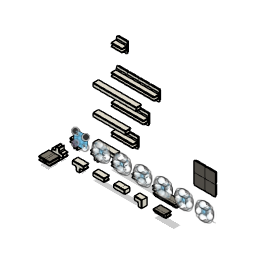
neogrid-03-master-file (Autodesk Fusion 360 design; units mm, degrees)
Autodesk Fusion 360 part; units mm, degrees
ref_plane "WorkPlane1" through (0, 0, 0) normal (0, 0, 1) x (1, 0, 0) in component "Gridfinity bin 1x1x1"
sketch "Sketch1" plane through (0, 0, 0) normal (0, 0, 1) x (1, 0, 0) in component "Gridfinity bin 1x1x1"
  line L0 (0, 0) -> (41.5, 0)
  line L1 (41.5, 0) -> (41.5, 41.5)
  line L2 (41.5, 41.5) -> (0, 41.5)
  line L3 (0, 41.5) -> (0, 0)
  dimension "d2" = 41.5
  dimension "d3" = 41.5
  constraint horizontal L0
  constraint vertical L1
  constraint horizontal L2
  constraint vertical L3
  constraint coincident L0.start L3
  constraint coincident L3.end L0
  measures "d2" horizontal distance of L0.start L0.end
  measures "d3" vertical distance of L0.end L1.end
extrude "Extrude1" add sketch "Sketch1" against normal blind 2.15 makes body 1 in component "Gridfinity bin 1x1x1"
fillet "Fillet1" radius 3.75 8 edges at (0, 0, -1.075) (41.5, 0, -1.075) (41.5, 0, -1.075) (41.5, 41.5, -1.075) (41.5, 41.5, -1.075) (0, 41.5, -1.075) (0, 41.5, -1.075) (0, 0, -1.075) on bodies 1 in component "Gridfinity bin 1x1x1"
chamfer "Chamfer1" distance 2.15 angle 45 8 edges at (1.0983, 40.4017, -2.15) (0, 20.75, -2.15) (1.0983, 1.0983, -2.15) (20.75, 0, -2.15) (40.4017, 1.0983, -2.15) (41.5, 20.75, -2.15) (40.4017, 40.4017, -2.15) (20.75, 41.5, -2.15) on bodies 1 in component "Gridfinity bin 1x1x1"
extrude "Extrude2" add 1 faces at (14.5499, 26.4167, -2.15) along direction (0, 0, -1) blind 2.6 on bodies 1 bodies 1 in component "Gridfinity bin 1x1x1"
chamfer "Chamfer2" distance 0.8 angle 45 8 edges at (2.6186, 38.8814, -4.75) (20.75, 39.35, -4.75) (38.8814, 38.8814, -4.75) (39.35, 20.75, -4.75) (38.8814, 2.6186, -4.75) (20.75, 2.15, -4.75) (2.6186, 2.6186, -4.75) (2.15, 20.75, -4.75) on bodies 1 in component "Gridfinity bin 1x1x1"
pattern_linear "R-Pattern1" count 1 spacing 42 along (1, 0, 0) of bodies 1 merged in component "Gridfinity bin 1x1x1"
sketch "Sketch2" plane through (0, 0, 0) normal (0, 0, 1) x (1, 0, 0) in component "Gridfinity bin 1x1x1"
  line L0 (0, 0) -> (41.5, 0)
  line L1 (41.5, 0) -> (41.5, 41.5)
  line L2 (41.5, 41.5) -> (0, 41.5)
  line L3 (0, 41.5) -> (0, 0)
  dimension "d16" = 41.5
  dimension "d17" = 41.5
  constraint horizontal L0
  constraint vertical L1
  constraint horizontal L2
  constraint vertical L3
  constraint coincident L0.start L3
  constraint coincident L3.end L0
  measures "d16" horizontal distance of L0.start L0.end
  measures "d17" vertical distance of L0.end L1.end
extrude "Extrude3" add sketch "Sketch2" along normal blind 2.25 separate body makes body 2 in component "Gridfinity bin 1x1x1"
fillet "Fillet2" radius 3.75 8 edges at (0, 41.5, 1.125) (41.5, 41.5, 1.125) (0, 0, 1.125) (0, 41.5, 1.125) (41.5, 41.5, 1.125) (41.5, 0, 1.125) (41.5, 0, 1.125) (0, 0, 1.125) on bodies 2 in component "Gridfinity bin 1x1x1"
combine "Combine1" operation add target body 2 tool bodies 1 1 in component "Gridfinity bin 1x1x1"
sketch "Master Dimensions" plane through (0, 0, 2.25) normal (0, 0, 1) x (1, 0, 0) in component "Gridfinity bin 1x1x1"
  arc A0 (37.75, 0) -> (41.5, 3.75) centre (37.75, 3.75) ccw
  line L0 (41.5, 3.75) -> (41.5, 37.75)
  arc A1 (41.5, 37.75) -> (37.75, 41.5) centre (37.75, 37.75) ccw
  line L1 (37.75, 41.5) -> (3.75, 41.5)
  arc A2 (3.75, 41.5) -> (0, 37.75) centre (3.75, 37.75) ccw
  line L2 (0, 37.75) -> (0, 3.75)
  arc A3 (0, 3.75) -> (3.75, 0) centre (3.75, 3.75) ccw
  line L3 (3.75, 0) -> (37.75, 0)
  line L4 (3.75, 41.5) -> (37.75, 41.5)
  line L5 (41.5, 37.75) -> (41.5, 3.75)
  line L6 (37.75, 0) -> (3.75, 0)
  line L7 (0, 3.75) -> (0, 37.75)
  arc A4 (3.75, 41.5) -> (0, 37.75) centre (3.75, 37.75) ccw
  arc A5 (41.5, 37.75) -> (37.75, 41.5) centre (37.75, 37.75) ccw
  arc A6 (0, 3.75) -> (3.75, 0) centre (3.75, 3.75) ccw
  arc A7 (37.75, 0) -> (41.5, 3.75) centre (37.75, 3.75) ccw
  line L8 (20.75, 41.5) -> (25, 41.5)
  line L9 (25, 41.5) -> (25, 0)
  line L10 (25, 0) -> (20.75, 0)
  line L11 (20.75, 0) -> (20.75, 41.5)
  line L12 (0, 20.75) -> (41.5, 20.75)
  line L13 (41.5, 20.75) -> (41.5, 25)
  line L14 (41.5, 25) -> (0, 25)
  line L15 (0, 25) -> (0, 20.75)
  line L16 (0, 20.75) -> (41.5, 20.75)
  line L17 (41.5, 20.75) -> (41.5, 16.5)
  line L18 (0, 16.5) -> (0, 20.75)
  line L19 (41.5, 16.5) -> (0, 16.5)
  line L20 (20.75, 0) -> (20.75, 41.5)
  line L21 (20.75, 41.5) -> (16.5, 41.5)
  line L22 (16.5, 0) -> (20.75, 0)
  line L23 (16.5, 41.5) -> (16.5, 0)
  line L24 (25, 41.5) -> (28, 41.5)
  line L25 (28, 41.5) -> (28, 0)
  line L26 (28, 0) -> (25, 0)
  line L27 (25, 0) -> (25, 41.5)
  line L28 (41.5, 25) -> (0, 25)
  line L29 (0, 25) -> (0, 28)
  line L30 (0, 28) -> (41.5, 28)
  line L31 (41.5, 28) -> (41.5, 25)
  line L32 (16.5, 41.5) -> (13.5, 41.5)
  line L33 (13.5, 0) -> (16.5, 0)
  line L34 (16.5, 0) -> (16.5, 41.5)
  line L35 (13.5, 41.5) -> (13.5, 0)
  line L36 (41.5, 16.5) -> (0, 16.5)
  line L37 (0, 16.5) -> (0, 13.5)
  line L38 (41.5, 13.5) -> (41.5, 16.5)
  line L39 (0, 13.5) -> (41.5, 13.5)
  line L40 (83.75, 41.5) -> (117.75, 41.5)
  arc A8 (83.75, 41.5) -> (80, 37.75) centre (83.75, 37.75) ccw
  line L41 (80, 3.75) -> (80, 37.75)
  arc A9 (80, 3.75) -> (83.75, 0) centre (83.75, 3.75) ccw
  line L42 (117.75, 0) -> (83.75, 0)
  arc A10 (117.75, 0) -> (121.5, 3.75) centre (117.75, 3.75) ccw
  line L43 (121.5, 37.75) -> (121.5, 3.75)
  arc A11 (121.5, 37.75) -> (117.75, 41.5) centre (117.75, 37.75) ccw
  line L44 (80, 28) -> (121.5, 28)
  line L45 (121.5, 25) -> (80, 25)
  line L46 (80, 20.75) -> (121.5, 20.75)
  line L47 (121.5, 16.5) -> (80, 16.5)
  line L48 (80, 13.5) -> (121.5, 13.5)
  line L49 (108, 41.5) -> (108, 0)
  line L50 (105, 41.5) -> (105, 0)
  line L51 (100.75, 0) -> (100.75, 41.5)
  line L52 (96.5, 41.5) -> (96.5, 0)
  line L53 (93.5, 41.5) -> (93.5, 0)
  line L54 (163.75, 41.5) -> (197.75, 41.5)
  arc A12 (163.75, 41.5) -> (160, 37.75) centre (163.75, 37.75) ccw
  line L55 (160, 3.75) -> (160, 37.75)
  arc A13 (160, 3.75) -> (163.75, 0) centre (163.75, 3.75) ccw
  line L56 (197.75, 0) -> (163.75, 0)
  arc A14 (197.75, 0) -> (201.5, 3.75) centre (197.75, 3.75) ccw
  line L57 (201.5, 37.75) -> (201.5, 3.75)
  arc A15 (201.5, 37.75) -> (197.75, 41.5) centre (197.75, 37.75) ccw
  line L58 (160, 28) -> (201.5, 28)
  line L59 (201.5, 25) -> (160, 25)
  line L60 (160, 20.75) -> (201.5, 20.75)
  line L61 (201.5, 16.5) -> (160, 16.5)
  line L62 (160, 13.5) -> (201.5, 13.5)
  line L63 (188, 41.5) -> (188, 0)
  line L64 (185, 41.5) -> (185, 0)
  line L65 (180.75, 0) -> (180.75, 41.5)
  line L66 (176.5, 41.5) -> (176.5, 0)
  line L67 (173.5, 41.5) -> (173.5, 0)
  line L68 (243.75, 41.5) -> (277.75, 41.5)
  arc A16 (243.75, 41.5) -> (240, 37.75) centre (243.75, 37.75) ccw
  line L69 (240, 3.75) -> (240, 37.75)
  arc A17 (240, 3.75) -> (243.75, 0) centre (243.75, 3.75) ccw
  line L70 (277.75, 0) -> (243.75, 0)
  arc A18 (277.75, 0) -> (281.5, 3.75) centre (277.75, 3.75) ccw
  line L71 (281.5, 37.75) -> (281.5, 3.75)
  arc A19 (281.5, 37.75) -> (277.75, 41.5) centre (277.75, 37.75) ccw
  line L72 (240, 28) -> (281.5, 28)
  line L73 (281.5, 25) -> (240, 25)
  line L74 (240, 20.75) -> (281.5, 20.75)
  line L75 (281.5, 16.5) -> (240, 16.5)
  line L76 (240, 13.5) -> (281.5, 13.5)
  line L77 (268, 41.5) -> (268, 0)
  line L78 (265, 41.5) -> (265, 0)
  line L79 (260.75, 0) -> (260.75, 41.5)
  line L80 (256.5, 41.5) -> (256.5, 0)
  line L81 (253.5, 41.5) -> (253.5, 0)
  line L82 (323.75, 41.5) -> (357.75, 41.5)
  arc A20 (323.75, 41.5) -> (320, 37.75) centre (323.75, 37.75) ccw
  line L83 (320, 3.75) -> (320, 37.75)
  arc A21 (320, 3.75) -> (323.75, 0) centre (323.75, 3.75) ccw
  line L84 (357.75, 0) -> (323.75, 0)
  arc A22 (357.75, 0) -> (361.5, 3.75) centre (357.75, 3.75) ccw
  line L85 (361.5, 37.75) -> (361.5, 3.75)
  arc A23 (361.5, 37.75) -> (357.75, 41.5) centre (357.75, 37.75) ccw
  line L86 (320, 28) -> (361.5, 28)
  line L87 (361.5, 25) -> (320, 25)
  line L88 (320, 20.75) -> (361.5, 20.75)
  line L89 (361.5, 16.5) -> (320, 16.5)
  line L90 (320, 13.5) -> (361.5, 13.5)
  line L91 (348, 41.5) -> (348, 0)
  line L92 (345, 41.5) -> (345, 0)
  line L93 (340.75, 0) -> (340.75, 41.5)
  line L94 (336.5, 41.5) -> (336.5, 0)
  line L95 (333.5, 41.5) -> (333.5, 0)
  line L96 (403.75, 41.5) -> (437.75, 41.5)
  arc A24 (403.75, 41.5) -> (400, 37.75) centre (403.75, 37.75) ccw
  line L97 (400, 3.75) -> (400, 37.75)
  arc A25 (400, 3.75) -> (403.75, 0) centre (403.75, 3.75) ccw
  line L98 (437.75, 0) -> (403.75, 0)
  arc A26 (437.75, 0) -> (441.5, 3.75) centre (437.75, 3.75) ccw
  line L99 (441.5, 37.75) -> (441.5, 3.75)
  arc A27 (441.5, 37.75) -> (437.75, 41.5) centre (437.75, 37.75) ccw
  line L100 (400, 28) -> (441.5, 28)
  line L101 (441.5, 25) -> (400, 25)
  line L102 (400, 20.75) -> (441.5, 20.75)
  line L103 (441.5, 16.5) -> (400, 16.5)
  line L104 (400, 13.5) -> (441.5, 13.5)
  line L105 (428, 41.5) -> (428, 0)
  line L106 (425, 41.5) -> (425, 0)
  line L107 (420.75, 0) -> (420.75, 41.5)
  line L108 (416.5, 41.5) -> (416.5, 0)
  line L109 (413.5, 41.5) -> (413.5, 0)
  line L110 (483.75, 41.5) -> (517.75, 41.5)
  arc A28 (483.75, 41.5) -> (480, 37.75) centre (483.75, 37.75) ccw
  line L111 (480, 3.75) -> (480, 37.75)
  arc A29 (480, 3.75) -> (483.75, 0) centre (483.75, 3.75) ccw
  line L112 (517.75, 0) -> (483.75, 0)
  arc A30 (517.75, 0) -> (521.5, 3.75) centre (517.75, 3.75) ccw
  line L113 (521.5, 37.75) -> (521.5, 3.75)
  arc A31 (521.5, 37.75) -> (517.75, 41.5) centre (517.75, 37.75) ccw
  line L114 (480, 28) -> (521.5, 28)
  line L115 (521.5, 25) -> (480, 25)
  line L116 (480, 20.75) -> (521.5, 20.75)
  line L117 (521.5, 16.5) -> (480, 16.5)
  line L118 (480, 13.5) -> (521.5, 13.5)
  line L119 (508, 41.5) -> (508, 0)
  line L120 (505, 41.5) -> (505, 0)
  line L121 (500.75, 0) -> (500.75, 41.5)
  line L122 (496.5, 41.5) -> (496.5, 0)
  line L123 (493.5, 41.5) -> (493.5, 0)
  point P0 (0, 41.5)
  point P1 (41.5, 41.5)
  dimension "d22" = 41.5
  dimension "d23" = 41.5
  dimension "d24" = 3.75
  dimension "d26" = 3.75
  dimension "d27" = 3.75
  dimension "d28" = 3.75
  dimension "d30" = 4.25
  dimension "d31" = 4.25
  dimension "d32" = 3
  dimension "d34" = 3
  dimension "d54" = 480
  dimension "d55" = 0
  constraint horizontal L4
  constraint vertical L5
  constraint horizontal L6
  constraint vertical L7
  constraint coincident P0 L4
  constraint coincident P0 L7
  constraint tangent L4 A4
  constraint tangent L7 A4
  constraint coincident P1 L4
  constraint coincident P1 L5
  constraint tangent L4 A5
  constraint tangent L5 A5
  constraint coincident origin L6
  constraint coincident origin L7
  constraint tangent L6 A6
  constraint tangent L7 A6
  constraint tangent L5 A7
  constraint tangent L6 A7
  constraint horizontal L8
  constraint vertical L9
  constraint horizontal L10
  constraint vertical L11
  constraint coincident L6 L9.end
  constraint midpoint L4 L8.start
  constraint horizontal L12
  constraint vertical L13
  constraint horizontal L14
  constraint vertical L15
  constraint midpoint L7 L12.start
  constraint symmetric L15.end L12 L16.start
  constraint symmetric L13.start L12 L16.end
  constraint symmetric L13.end L12 L17.end
  constraint symmetric L14.end L12 L18.start
  constraint symmetric L8.start L11 L20.end
  constraint symmetric L8.end L11 L21.end
  constraint symmetric L9.end L11 L22.start
  constraint symmetric L10.end L11 L20.start
  constraint horizontal L24
  constraint vertical L25
  constraint horizontal L26
  constraint vertical L27
  constraint horizontal L28
  constraint vertical L29
  constraint horizontal L30
  constraint vertical L31
  constraint symmetric L8.end L20 L21.end
  constraint symmetric L20 L24.end L32.end
  constraint symmetric L20 L25.end L33.start
  constraint symmetric L20 L9.end L22.start
  constraint symmetric L12 L14.end L18.start
  constraint symmetric L12 L29.end L37.end
  constraint symmetric L12 L30.end L38.start
  measures "d22" distance of P0 origin
  measures "d23" distance of P0 P1
  measures "d24" radius of A4
  measures "d26" radius of A5
  measures "d27" radius of A6
  measures "d28" radius of A7
  measures "d30" distance of L8.start L8.end
  measures "d31" distance of L12.start L14.end
  measures "d32" distance of L8.end L24.end
  measures "d34" distance of L13.end L30.end
pattern_linear "R-Pattern2" count 7 spacing 80 along (1, 0, 0) of bodies 2 makes body 3 at (105.1667, 15.0833, 2.25) makes body 4 at (185.1667, 15.0833, 2.25) makes body 5 at (265.1667, 15.0833, 2.25) makes body 6 at (345.1667, 15.0833, 2.25) makes body 7 at (425.1667, 15.0833, 2.25) makes body 8 at (505.1667, 15.0833, 2.25) in component "Gridfinity bin 1x1x1"
extrude "Extrude4" add sketch "Master Dimensions" along normal blind 21 contours L3 L6 L9 L25 L26 L27 L39 | L0 L5 L19 L25 L36 L38 L39 | L9 L19 L25 L27 L36 L39 | L3 L6 L23 L33 L34 L35 L39 | L0 L5 L14 L25 L28 L30 L31 | L19 L23 L34 L35 L36 L39 | L9 L14 L25 L27 L28 L30 | L2 L7 L19 L35 L36 L37 L39 | L1 L4 L9 L24 L25 L27 L30 | L14 L23 L28 L30 L34 L35 | L2 L7 L14 L28 L29 L30 L35 | L1 L4 L23 L30 L32 L34 L35 | L41 L44 L45 L53 | L44 L45 L52 L53 | L44 L45 L51 L52 | L44 L45 L50 L51 | L44 L45 L49 L50 | L41 L47 L48 L53 | L47 L48 L52 L53 | L43 L44 L45 L49 | L42 L48 L52 L53 | L47 L48 L49 L50 | L43 L47 L48 L49 | L42 L48 L49 L50 | L55 L58 L59 L67 | L58 L59 L66 L67 | L58 L59 L65 L66 | L58 L59 L64 L65 | L58 L59 L63 L64 | L55 L61 L62 L67 | L61 L62 L66 L67 | L57 L58 L59 L63 | L61 L62 L65 L66 | L61 L62 L64 L65 | L61 L62 L63 L64 | L57 L61 L62 L63 | L69 L72 L73 L81 | L72 L73 L80 L81 | L72 L73 L79 L80 | L72 L73 L78 L79 | L72 L73 L77 L78 | L69 L75 L76 L81 | L75 L76 L80 L81 | L71 L72 L73 L77 | L73 L74 L77 L78 | L75 L76 L79 L80 | L71 L73 L74 L77 | L74 L75 L77 L78 | L75 L76 L78 L79 | L71 L74 L75 L77 | L75 L76 L77 L78 | L71 L75 L76 L77 | L83 L86 L87 L95 | L86 L87 L94 L95 | L86 L87 L93 L94 | L86 L87 L92 L93 | L86 L87 L91 L92 | L83 L89 L90 L95 | L89 L90 L94 L95 | L87 L88 L91 L92 | L84 L90 L94 L95 | L88 L89 L91 L92 | L89 L90 L91 L92 | L84 L90 L91 L92 bodies 2 3 4 5 6 in component "Gridfinity bin 1x1x1"
chamfer "Chamfer3" distance 3 angle 45 4 edges at (28, 13.5, 12.75) (13.5, 13.5, 12.75) (28, 28, 12.75) (13.5, 28, 12.75) on bodies 2 3 6 in component "Gridfinity bin 1x1x1"
chamfer "Chamfer3" distance 3 angle 45 3 edges at (333.5, 13.5, 12.75) (108, 13.5, 12.75) (93.5, 13.5, 12.75) on bodies 2 3 6 in component "Gridfinity bin 1x1x1"
chamfer "Chamfer4" distance 3 angle 45 12 edges at (29.5, 12, 2.25) (36.25, 13.5, 2.25) (28, 5.25, 2.25) (5.25, 13.5, 2.25) (12, 12, 2.25) (13.5, 5.25, 2.25) (13.5, 36.25, 2.25) (12, 29.5, 2.25) (5.25, 28, 2.25) (36.25, 28, 2.25) (29.5, 29.5, 2.25) (28, 36.25, 2.25) on bodies 2 3 4 5 6 in component "Gridfinity bin 1x1x1"
chamfer "Chamfer4" distance 3 angle 45 16 edges at (260.75, 13.5, 2.25) (260.75, 28, 2.25) (332, 12, 2.25) (325.25, 13.5, 2.25) (333.5, 5.25, 2.25) (334, 28, 2.25) (348, 14, 2.25) (85.25, 13.5, 2.25) (116.25, 13.5, 2.25) (109.5, 12, 2.25) (108, 5.25, 2.25) (92, 12, 2.25) (93.5, 5.25, 2.25) (100.75, 28, 2.25) (180.75, 28, 2.25) (180.75, 13.5, 2.25) on bodies 2 3 4 5 6 in component "Gridfinity bin 1x1x1"
chamfer "Chamfer5" distance 1.5 angle 45 12 edges at (5.25, 13.5, 23.25) (12, 12, 23.25) (13.5, 5.25, 23.25) (28, 5.25, 23.25) (29.5, 12, 23.25) (36.25, 13.5, 23.25) (36.25, 28, 23.25) (29.5, 29.5, 23.25) (28, 36.25, 23.25) (12, 29.5, 23.25) (13.5, 36.25, 23.25) (5.25, 28, 23.25) on bodies 2 3 4 5 6 in component "Gridfinity bin 1x1x1"
chamfer "Chamfer5" distance 1.5 angle 45 17 edges at (260.75, 28, 23.25) (281.5, 20.75, 23.25) (260.75, 13.5, 23.25) (334, 28, 23.25) (348, 14, 23.25) (333.5, 5.25, 23.25) (332, 12, 23.25) (325.25, 13.5, 23.25) (85.25, 13.5, 23.25) (92, 12, 23.25) (93.5, 5.25, 23.25) (109.5, 12, 23.25) (116.25, 13.5, 23.25) (108, 5.25, 23.25) (100.75, 28, 23.25) (180.75, 28, 23.25) (180.75, 13.5, 23.25) on bodies 2 3 4 5 6 in component "Gridfinity bin 1x1x1"
extrude "Extrude5" add sketch "Master Dimensions" 1 faces at (99.3333, 22.1667, 2.25) along normal blind 21 from surface at 70 separate body contours L3 L6 L9 L25 L26 L27 L39 | L0 L5 L19 L25 L36 L38 L39 | L3 L6 L9 L10 L11 L20 L27 L39 | L9 L19 L25 L27 L36 L39 | L0 L5 L12 L16 L17 L19 L25 L36 | L3 L6 L11 L20 L22 L23 L34 L39 | L9 L11 L19 L20 L27 L36 L39 | L9 L12 L16 L19 L25 L27 L36 | L0 L5 L12 L13 L14 L16 L25 L28 | L3 L6 L23 L33 L34 L35 L39 | L11 L19 L20 L23 L34 L36 L39 | L9 L11 L12 L16 L19 L20 L27 L36 | L9 L12 L14 L16 L25 L27 L28 | L0 L5 L14 L25 L28 L30 L31 | L19 L23 L34 L35 L36 L39 | L11 L12 L16 L19 L20 L23 L34 L36 | L9 L11 L12 L14 L16 L20 L27 L28 | L9 L14 L25 L27 L28 L30 | L2 L7 L19 L35 L36 L37 L39 | L12 L16 L19 L23 L34 L35 L36 | L11 L12 L14 L16 L20 L23 L28 L34 | L9 L11 L14 L20 L27 L28 L30 | L1 L4 L9 L24 L25 L27 L30 | L2 L7 L12 L16 L18 L19 L35 L36 | L12 L14 L16 L23 L28 L34 L35 | L11 L14 L20 L23 L28 L30 L34 | L1 L4 L8 L9 L11 L20 L27 L30 | L2 L7 L12 L14 L15 L16 L28 L35 | L14 L23 L28 L30 L34 L35 | L1 L4 L11 L20 L21 L23 L30 L34 | L2 L7 L14 L28 L29 L30 L35 | L1 L4 L23 L30 L32 L34 L35 | L41 L44 L45 L53 | L44 L45 L52 L53 | L44 L45 L51 L52 | L44 L45 L50 L51 | L44 L45 L49 L50 | L41 L47 L48 L53 | L47 L48 L52 L53 | L43 L44 L45 L49 | L42 L48 L52 L53 | L47 L48 L49 L50 | L43 L47 L48 L49 | L42 L48 L49 L50 | L55 L58 L59 L67 | L58 L59 L66 L67 | L58 L59 L65 L66 | L55 L59 L60 L67 | L59 L60 L66 L67 | L58 L59 L64 L65 | L59 L60 L65 L66 | L55 L60 L61 L67 | L60 L61 L66 L67 | L58 L59 L63 L64 | L59 L60 L64 L65 | L60 L61 L65 L66 | L55 L61 L62 L67 | L61 L62 L66 L67 | L57 L58 L59 L63 | L59 L60 L63 L64 | L60 L61 L64 L65 | L61 L62 L65 L66 | L57 L59 L60 L63 | L60 L61 L63 L64 | L61 L62 L64 L65 | L57 L60 L61 L63 | L61 L62 L63 L64 | L57 L61 L62 L63 | L69 L72 L73 L81 | L72 L73 L80 L81 | L72 L73 L79 L80 | L69 L73 L74 L81 | L73 L74 L80 L81 | L72 L73 L78 L79 | L73 L74 L79 L80 | L69 L74 L75 L81 | L74 L75 L80 L81 | L72 L73 L77 L78 | L73 L74 L78 L79 | L74 L75 L79 L80 | L69 L75 L76 L81 | L75 L76 L80 L81 | L71 L72 L73 L77 | L73 L74 L77 L78 | L74 L75 L78 L79 | L75 L76 L79 L80 | L71 L73 L74 L77 | L74 L75 L77 L78 | L75 L76 L78 L79 | L71 L74 L75 L77 | L75 L76 L77 L78 | L71 L75 L76 L77 | L83 L86 L87 L95 | L86 L87 L94 L95 | L86 L87 L93 L94 | L83 L87 L88 L95 | L87 L88 L94 L95 | L86 L87 L92 L93 | L87 L88 L93 L94 | L83 L88 L89 L95 | L88 L89 L94 L95 | L86 L87 L91 L92 | L87 L88 L92 L93 | L88 L89 L93 L94 | L83 L89 L90 L95 | L89 L90 L94 L95 | L87 L88 L91 L92 | L88 L89 L92 L93 | L89 L90 L93 L94 | L84 L90 L94 L95 | L88 L89 L91 L92 | L89 L90 L92 L93 | L84 L90 L93 L94 | L89 L90 L91 L92 | L84 L90 L92 L93 | L84 L90 L91 L92 | L97 L100 L101 L109 | L100 L101 L108 L109 | L100 L101 L107 L108 | L97 L101 L102 L109 | L101 L102 L108 L109 | L100 L101 L106 L107 | L101 L102 L107 L108 | L97 L102 L103 L109 | L102 L103 L108 L109 | L100 L101 L105 L106 | L101 L102 L106 L107 | L102 L103 L107 L108 | L97 L103 L104 L109 | L103 L104 L108 L109 | L99 L100 L101 L105 | L101 L102 L105 L106 | L102 L103 L106 L107 | L103 L104 L107 L108 | L99 L101 L102 L105 | L102 L103 L105 L106 | L103 L104 L106 L107 | L99 L102 L103 L105 | L103 L104 L105 L106 | L99 L103 L104 L105 on bodies 3 makes body 9 at (18.3333, 18.3333, 72.25) makes body 10 at (343.1667, 13.8333, 72.25) makes body 11 at (253.8333, 13.5, 86.25) makes body 12 at (93.8333, 28, 86.25) makes body 13 at (173.8333, 13.5, 86.25) makes body 14 at (413.8333, 13.5, 86.25) in component "Gridfinity bin 1x1x1"
extrude "Extrude6" cut sketch "Master Dimensions" along normal blind 18 from surface at 70 contours L3 L6 L9 L10 L11 L20 L27 L39 | L0 L5 L12 L16 L17 L19 L25 L36 | L3 L6 L11 L20 L22 L23 L34 L39 | L9 L11 L19 L20 L27 L36 L39 | L9 L12 L16 L19 L25 L27 L36 | L0 L5 L12 L13 L14 L16 L25 L28 | L11 L19 L20 L23 L34 L36 L39 | L9 L11 L12 L16 L19 L20 L27 L36 | L9 L12 L14 L16 L25 L27 L28 | L11 L12 L16 L19 L20 L23 L34 L36 | L9 L11 L12 L14 L16 L20 L27 L28 | L12 L16 L19 L23 L34 L35 L36 | L11 L12 L14 L16 L20 L23 L28 L34 | L9 L11 L14 L20 L27 L28 L30 | L2 L7 L12 L16 L18 L19 L35 L36 | L12 L14 L16 L23 L28 L34 L35 | L11 L14 L20 L23 L28 L30 L34 | L1 L4 L8 L9 L11 L20 L27 L30 | L2 L7 L12 L14 L15 L16 L28 L35 | L1 L4 L11 L20 L21 L23 L30 L34 | L41 L45 L46 L53 | L45 L46 L52 L53 | L45 L46 L51 L52 | L41 L46 L47 L53 | L46 L47 L52 L53 | L45 L46 L50 L51 | L46 L47 L51 L52 | L45 L46 L49 L50 | L46 L47 L50 L51 | L47 L48 L51 L52 | L43 L45 L46 L49 | L46 L47 L49 L50 | L47 L48 L50 L51 | L42 L48 L51 L52 | L43 L46 L47 L49 | L42 L48 L50 L51 | L55 L59 L60 L67 | L59 L60 L66 L67 | L59 L60 L65 L66 | L55 L60 L61 L67 | L60 L61 L66 L67 | L59 L60 L64 L65 | L60 L61 L65 L66 | L59 L60 L63 L64 | L60 L61 L64 L65 | L57 L59 L60 L63 | L60 L61 L63 L64 | L57 L60 L61 L63 | L69 L73 L74 L81 | L73 L74 L80 L81 | L73 L74 L79 L80 | L69 L74 L75 L81 | L74 L75 L80 L81 | L73 L74 L78 L79 | L74 L75 L79 L80 | L74 L75 L78 L79 | L83 L87 L88 L95 | L87 L88 L94 L95 | L87 L88 L93 L94 | L83 L88 L89 L95 | L88 L89 L94 L95 | L87 L88 L92 L93 | L88 L89 L93 L94 | L88 L89 L92 L93 | L89 L90 L93 L94 | L89 L90 L92 L93 | L84 L90 L93 L94 | L84 L90 L92 L93 | L97 L101 L102 L109 | L101 L102 L108 L109 | L101 L102 L107 L108 | L97 L102 L103 L109 | L102 L103 L108 L109 | L101 L102 L106 L107 | L102 L103 L107 L108 | L101 L102 L105 L106 | L102 L103 L106 L107 | L99 L101 L102 L105 | L102 L103 L105 L106 | L99 L102 L103 L105 bodies 14 9 13 10 12 11 in component "Gridfinity bin 1x1x1"
chamfer "Chamfer6" distance 3 angle 45 4 edges at (28, 28, 82.75) (13.5, 28, 82.75) (13.5, 13.5, 82.75) (28, 13.5, 82.75) on bodies 9 10 12 in component "Gridfinity bin 1x1x1"
chamfer "Chamfer6" distance 3 angle 45 3 edges at (333.5, 13.5, 82.75) (108, 13.5, 82.75) (93.5, 13.5, 82.75) on bodies 9 10 12 in component "Gridfinity bin 1x1x1"
chamfer "Chamfer7" distance 1.5 angle 45 12 edges at (13.5, 36.25, 93.25) (12, 29.5, 93.25) (5.25, 28, 93.25) (5.25, 13.5, 93.25) (12, 12, 93.25) (13.5, 5.25, 93.25) (28, 5.25, 93.25) (29.5, 12, 93.25) (36.25, 13.5, 93.25) (36.25, 28, 93.25) (29.5, 29.5, 93.25) (28, 36.25, 93.25) on bodies 9 10 11 12 13 14 in component "Gridfinity bin 1x1x1"
chamfer "Chamfer7" distance 1.5 angle 45 17 edges at (180.75, 28, 93.25) (180.75, 13.5, 93.25) (334, 28, 93.25) (348, 14, 93.25) (333.5, 5.25, 93.25) (332, 12, 93.25) (325.25, 13.5, 93.25) (260.75, 28, 93.25) (260.75, 13.5, 93.25) (281.5, 20.75, 93.25) (116.25, 13.5, 93.25) (109.5, 12, 93.25) (108, 5.25, 93.25) (85.25, 13.5, 93.25) (93.5, 5.25, 93.25) (92, 12, 93.25) (100.75, 28, 93.25) on bodies 9 10 11 12 13 14 in component "Gridfinity bin 1x1x1"
chamfer "Chamfer7" distance 1.5 angle 45 1 edges at (420.75, 28, 93.25) on bodies 9 10 11 12 13 14 in component "Gridfinity bin 1x1x1"
chamfer "Chamfer8" distance 1.5 angle 45 12 edges at (28, 36.25, 72.25) (29.5, 29.5, 72.25) (36.25, 28, 72.25) (12, 29.5, 72.25) (5.25, 28, 72.25) (13.5, 36.25, 72.25) (12, 12, 72.25) (13.5, 5.25, 72.25) (5.25, 13.5, 72.25) (29.5, 12, 72.25) (36.25, 13.5, 72.25) (28, 5.25, 72.25) on bodies 9 in component "Gridfinity bin 1x1x1"
sketch "Sketch1 (2)" plane through (441.5, 0, 0) normal (1, 0, 0) x (0, 0, -1)
  line L0 (-91.75, 28) -> (-93.25, 26.5)
  line L1 (-93.25, 26.5) -> (-93.25, 13.5)
  line L2 (-93.25, 13.5) -> (-72.25, 13.5)
  line L3 (-72.25, 13.5) -> (-72.25, 16.5)
  line L4 (-72.25, 16.5) -> (-90.25, 16.5)
  line L5 (-90.25, 16.5) -> (-90.25, 25)
  line L6 (-90.25, 25) -> (-72.25, 25)
  line L7 (-72.25, 25) -> (-72.25, 28)
  line L8 (-72.25, 28) -> (-91.75, 28)
  line L9 (-93.25, 13.5) -> (-101.6216, 28)
  line L10 (-101.6216, 28) -> (-91.75, 28)
  dimension "d76" = 30
  constraint coincident L1.end L2.start
  constraint coincident L0.start L8.end
  constraint collinear L8 L10
  measures "d76" angle of L1 L9
extrude "Extrude7" add sketch "Sketch1 (2)" against normal up to surface (41.5 mm away) contours L0 L1 L9 L10 bodies 14 in component "Gridfinity bin 1x1x1"
chamfer "Chamfer9" distance 1.5 angle 45 1 edges at (420.75, 28, 101.6216) on bodies 14 in component "Gridfinity bin 1x1x1"
pattern_linear "R-Pattern3" count 2 spacing 55 along (0, 1, 0) of bodies 14 makes body 15 in component "Gridfinity bin 1x1x1"
extrude "Extrude8" add 1 faces at (441.5, 77.7337, 93.7905) along direction (1, 0, 0) blind 41.5 on bodies 15 bodies 15 in component "Gridfinity bin 1x1x1"
pattern_linear "R-Pattern4" count 5 spacing 100 along (0, 1, 0) of bodies 4 makes body 16 at (174.8165, 115.0833, -4.75) makes body 17 at (174.8165, 215.0833, -4.75) makes body 18 at (174.8165, 315.0833, -4.75) makes body 19 at (174.8165, 415.0833, -4.75) in component "Gridfinity bin 1x1x1"
pattern_linear "R-Pattern5" count 2 spacing 41.5 along (1, 0, 0) of bodies 16 makes body 20 in component "Gridfinity bin 1x1x1"
combine "Combine2" operation add target body 16 tool bodies 20 in component "Gridfinity bin 1x1x1"
sketch "Sketch3" plane through (160, 0, 0) normal (-1, 0, 0) x (0, 0, 1)
  line L0 (21.75, 113.5) -> (23.25, 115)
  line L1 (23.25, 115) -> (23.25, 116.5)
  line L2 (23.25, 116.5) -> (2.25, 116.5)
  line L3 (2.25, 116.5) -> (2.25, 125)
  line L4 (2.25, 125) -> (23.25, 125)
  line L5 (23.25, 125) -> (23.25, 126.5)
  line L6 (23.25, 126.5) -> (21.75, 128)
  line L7 (21.75, 128) -> (5.25, 128)
  line L8 (5.25, 128) -> (2.25, 131)
  line L9 (2.25, 131) -> (2.25, 137.75)
  line L10 (2.25, 137.75) -> (0, 137.75)
  line L11 (0, 137.75) -> (0, 103.75)
  line L12 (0, 103.75) -> (2.25, 103.75)
  line L13 (2.25, 103.75) -> (2.25, 110.5)
  line L14 (2.25, 110.5) -> (5.25, 113.5)
  line L15 (5.25, 113.5) -> (21.75, 113.5)
  line L16 (0, 100) -> (2.25, 100)
  line L17 (2.25, 100) -> (2.25, 141.5)
  line L18 (2.25, 141.5) -> (0, 141.5)
  line L19 (0, 141.5) -> (0, 100)
  line L20 (2.25, 141.5) -> (0, 141.5)
  line L21 (0, 100) -> (2.25, 100)
  constraint horizontal L16
  constraint vertical L17
  constraint horizontal L18
  constraint vertical L19
  constraint collinear L18 L20
  constraint collinear L16 L21
extrude "Extrude9" add sketch "Sketch3" against normal blind 30 from surface at -30 contours L12 L16 L17 L19 L21 | L10 L17 L18 L19 L20 bodies 16 in component "Gridfinity bin 1x1x1"
pattern_linear "R-Pattern6" count 3 spacing 41.5 along (1, 0, 0) of bodies 17 makes body 21 at (216.3165, 215.0833, -4.75) makes body 22 at (257.8165, 215.0833, -4.75) in component "Gridfinity bin 1x1x1"
pattern_linear "R-Pattern7" count 4 spacing 41.5 along (1, 0, 0) of bodies 18 makes body 23 at (216.3165, 315.0833, -4.75) makes body 24 at (257.8165, 315.0833, -4.75) makes body 25 at (299.3165, 315.0833, -4.75) in component "Gridfinity bin 1x1x1"
combine "Combine3" operation add target body 17 tool bodies 21 22 in component "Gridfinity bin 1x1x1"
combine "Combine4" operation add target body 18 tool bodies 23 24 25 in component "Gridfinity bin 1x1x1"
sketch "Sketch4" plane through (160, 0, 0) normal (-1, 0, 0) x (0, 0, 1)
  line L0 (21.75, 213.5) -> (23.25, 215)
  line L1 (23.25, 215) -> (23.25, 216.5)
  line L2 (23.25, 216.5) -> (2.25, 216.5)
  line L3 (2.25, 216.5) -> (2.25, 225)
  line L4 (2.25, 225) -> (23.25, 225)
  line L5 (23.25, 225) -> (23.25, 226.5)
  line L6 (23.25, 226.5) -> (21.75, 228)
  line L7 (21.75, 228) -> (5.25, 228)
  line L8 (5.25, 228) -> (2.25, 231)
  line L9 (2.25, 231) -> (2.25, 237.75)
  line L10 (2.25, 237.75) -> (0, 237.75)
  line L11 (0, 237.75) -> (0, 203.75)
  line L12 (0, 203.75) -> (2.25, 203.75)
  line L13 (2.25, 203.75) -> (2.25, 210.5)
  line L14 (2.25, 210.5) -> (5.25, 213.5)
  line L15 (5.25, 213.5) -> (21.75, 213.5)
  line L16 (0, 241.5) -> (2.25, 241.5)
  line L17 (2.25, 241.5) -> (2.25, 200)
  line L18 (2.25, 200) -> (0, 200)
  line L19 (0, 200) -> (0, 241.5)
  line L20 (0, 200) -> (2.25, 200)
  line L21 (2.25, 241.5) -> (0, 241.5)
  constraint horizontal L16
  constraint vertical L17
  constraint horizontal L18
  constraint vertical L19
  constraint collinear L3 L17
  constraint collinear L18 L20
  constraint collinear L16 L21
  constraint collinear L11 L19
extrude "Extrude10" add sketch "Sketch4" against normal blind 74 from surface at -30 contours L12 L17 L18 L19 L20 | L10 L16 L17 L19 L21 bodies 17 in component "Gridfinity bin 1x1x1"
sketch "Sketch5" plane through (160, 0, 0) normal (-1, 0, 0) x (0, 0, 1)
  line L0 (21.75, 313.5) -> (23.25, 315)
  line L1 (23.25, 315) -> (23.25, 316.5)
  line L2 (23.25, 316.5) -> (2.25, 316.5)
  line L3 (2.25, 316.5) -> (2.25, 325)
  line L4 (2.25, 325) -> (23.25, 325)
  line L5 (23.25, 325) -> (23.25, 326.5)
  line L6 (23.25, 326.5) -> (21.75, 328)
  line L7 (21.75, 328) -> (5.25, 328)
  line L8 (5.25, 328) -> (2.25, 331)
  line L9 (2.25, 331) -> (2.25, 337.75)
  line L10 (2.25, 337.75) -> (0, 337.75)
  line L11 (0, 337.75) -> (0, 303.75)
  line L12 (0, 303.75) -> (2.25, 303.75)
  line L13 (2.25, 303.75) -> (2.25, 310.5)
  line L14 (2.25, 310.5) -> (5.25, 313.5)
  line L15 (5.25, 313.5) -> (21.75, 313.5)
  line L16 (0, 341.5) -> (2.25, 341.5)
  line L17 (2.25, 341.5) -> (2.25, 300)
  line L18 (2.25, 300) -> (0, 300)
  line L19 (0, 300) -> (0, 341.5)
  line L20 (0, 300) -> (2.25, 300)
  line L21 (2.25, 341.5) -> (0, 341.5)
  constraint horizontal L16
  constraint vertical L17
  constraint horizontal L18
  constraint vertical L19
  constraint collinear L18 L20
  constraint collinear L16 L21
extrude "Extrude11" add sketch "Sketch5" against normal blind 106 from surface at -30 contours L12 L17 L18 L19 L20 | L10 L16 L17 L19 L21 bodies 18 in component "Gridfinity bin 1x1x1"
pattern_linear "R-Pattern8" count 4 spacing 100 along (0, 1, 0) of bodies 13 makes body 26 at (173.8333, 128, 78.75) makes body 27 at (173.8333, 228, 78.75) makes body 28 at (173.8333, 328, 78.75) in component "Gridfinity bin 1x1x1"
extrude "Extrude12" add 1 faces at (201.5, 127, 84.75) along direction (1, 0, 0) blind 41.5 on bodies 26 bodies 26 in component "Gridfinity bin 1x1x1"
extrude "Extrude13" add 1 faces at (201.5, 214.5, 84.75) along direction (1, 0, 0) blind 83 on bodies 27 bodies 27 in component "Gridfinity bin 1x1x1"
extrude "Extrude14" add 1 faces at (201.5, 314.5, 84.75) along direction (1, 0, 0) blind 124.5 on bodies 28 bodies 28 in component "Gridfinity bin 1x1x1"
ref_plane "WorkPlane1" through (0, 0, 0) normal (0, 0, 1) x (1, 0, 0) in component "Neogrid - Base Cover 2x2"
sketch "Sketch1 (3)" plane through (0, 0, 0) normal (0, 0, 1) x (1, 0, 0) in component "Neogrid - Base Cover 2x2"
  line L0 (0, 0) -> (41.5, 0)
  line L1 (41.5, 0) -> (41.5, 41.5)
  line L2 (41.5, 41.5) -> (0, 41.5)
  line L3 (0, 41.5) -> (0, 0)
  dimension "d113" = 41.5
  dimension "d114" = 41.5
  constraint horizontal L0
  constraint vertical L1
  constraint horizontal L2
  constraint vertical L3
  constraint coincident L0.start L3
  constraint coincident L3.end L0
  measures "d113" horizontal distance of L0.start L0.end
  measures "d114" vertical distance of L0.end L1.end
extrude "Extrude1'" add sketch "Sketch1 (3)" against normal blind 2.15 separate body makes body 29 in component "Neogrid - Base Cover 2x2"
fillet "Fillet1'" radius 3.75 8 edges at (0, 0, -1.075) (41.5, 0, -1.075) (41.5, 0, -1.075) (41.5, 41.5, -1.075) (41.5, 41.5, -1.075) (0, 41.5, -1.075) (0, 41.5, -1.075) (0, 0, -1.075) on bodies 29 in component "Neogrid - Base Cover 2x2"
chamfer "Chamfer1'" distance 2.15 angle 45 8 edges at (1.0983, 40.4017, -2.15) (0, 20.75, -2.15) (1.0983, 1.0983, -2.15) (20.75, 0, -2.15) (40.4017, 1.0983, -2.15) (41.5, 20.75, -2.15) (40.4017, 40.4017, -2.15) (20.75, 41.5, -2.15) on bodies 29 in component "Neogrid - Base Cover 2x2"
extrude "Extrude2'" add 1 faces at (14.5499, 26.4167, -2.15) along direction (0, 0, -1) blind 2.6 on bodies 29 bodies 29 in component "Neogrid - Base Cover 2x2"
chamfer "Chamfer2'" distance 0.8 angle 45 8 edges at (2.6186, 38.8814, -4.75) (20.75, 39.35, -4.75) (38.8814, 38.8814, -4.75) (39.35, 20.75, -4.75) (38.8814, 2.6186, -4.75) (20.75, 2.15, -4.75) (2.6186, 2.6186, -4.75) (2.15, 20.75, -4.75) on bodies 29 in component "Neogrid - Base Cover 2x2"
pattern_linear "R-Pattern1'" count 2 spacing 42 along (1, 0, 0) count 2 spacing 42 along (0, 1, 0) of bodies 29 makes body 30 at (68.4167, 16.3333, 0) makes body 31 at (25.1667, 57.0833, 0) makes body 32 at (68.4167, 58.3333, 0) in component "Neogrid - Base Cover 2x2"
sketch "Sketch2 (2)" plane through (0, 0, 0) normal (0, 0, 1) x (1, 0, 0) in component "Neogrid - Base Cover 2x2"
  line L0 (0, 0) -> (83.5, 0)
  line L1 (83.5, 0) -> (83.5, 83.5)
  line L2 (83.5, 83.5) -> (0, 83.5)
  line L3 (0, 83.5) -> (0, 0)
  dimension "d127" = 83.5
  dimension "d128" = 83.5
  constraint horizontal L0
  constraint vertical L1
  constraint horizontal L2
  constraint vertical L3
  constraint coincident L0.start L3
  constraint coincident L3.end L0
  measures "d127" horizontal distance of L0.start L0.end
  measures "d128" vertical distance of L0.end L1.end
extrude "Extrude3'" add sketch "Sketch2 (2)" along normal blind 2.25 separate body makes body 33 in component "Neogrid - Base Cover 2x2"
fillet "Fillet2'" radius 3.75 8 edges at (0, 83.5, 1.125) (83.5, 83.5, 1.125) (83.5, 83.5, 1.125) (83.5, 0, 1.125) (83.5, 0, 1.125) (0, 0, 1.125) (0, 0, 1.125) (0, 83.5, 1.125) on bodies 33 in component "Neogrid - Base Cover 2x2"
combine "Combine1'" operation add target body 33 tool bodies 29 30 31 32 29 in component "Neogrid - Base Cover 2x2"
move_body "Move1" bodies 33 to x (1, 0, 0) y (0, 1, 0) z (0, 0, 1) at (460, 90, 0) in component "Neogrid - Base Cover 2x2"
ref_plane "WorkPlane1" through (0, 0, 0) normal (0, 0, 1) x (1, 0, 0) in component "Neogrid - Base Cover 2x1"
sketch "Sketch1 (4)" plane through (0, 0, 0) normal (0, 0, 1) x (1, 0, 0) in component "Neogrid - Base Cover 2x1"
  line L0 (0, 0) -> (41.5, 0)
  line L1 (41.5, 0) -> (41.5, 41.5)
  line L2 (41.5, 41.5) -> (0, 41.5)
  line L3 (0, 41.5) -> (0, 0)
  dimension "d134" = 41.5
  dimension "d135" = 41.5
  constraint horizontal L0
  constraint vertical L1
  constraint horizontal L2
  constraint vertical L3
  constraint coincident L0.start L3
  constraint coincident L3.end L0
  measures "d134" horizontal distance of L0.start L0.end
  measures "d135" vertical distance of L0.end L1.end
extrude "Extrude1''" add sketch "Sketch1 (4)" against normal blind 2.15 separate body makes body 34 in component "Neogrid - Base Cover 2x1"
fillet "Fillet1''" radius 3.75 8 edges at (0, 0, -1.075) (41.5, 0, -1.075) (41.5, 0, -1.075) (41.5, 41.5, -1.075) (41.5, 41.5, -1.075) (0, 41.5, -1.075) (0, 41.5, -1.075) (0, 0, -1.075) on bodies 34 in component "Neogrid - Base Cover 2x1"
chamfer "Chamfer1''" distance 2.15 angle 45 8 edges at (1.0983, 40.4017, -2.15) (0, 20.75, -2.15) (1.0983, 1.0983, -2.15) (20.75, 0, -2.15) (40.4017, 1.0983, -2.15) (41.5, 20.75, -2.15) (40.4017, 40.4017, -2.15) (20.75, 41.5, -2.15) on bodies 34 in component "Neogrid - Base Cover 2x1"
extrude "Extrude2''" add 1 faces at (14.5499, 26.4167, -2.15) along direction (0, 0, -1) blind 2.6 on bodies 34 bodies 34 in component "Neogrid - Base Cover 2x1"
chamfer "Chamfer2''" distance 0.8 angle 45 8 edges at (2.6186, 38.8814, -4.75) (20.75, 39.35, -4.75) (38.8814, 38.8814, -4.75) (39.35, 20.75, -4.75) (38.8814, 2.6186, -4.75) (20.75, 2.15, -4.75) (2.6186, 2.6186, -4.75) (2.15, 20.75, -4.75) on bodies 34 in component "Neogrid - Base Cover 2x1"
pattern_linear "R-Pattern1''" count 2 spacing 42 along (1, 0, 0) of bodies 34 makes body 35 in component "Neogrid - Base Cover 2x1"
sketch "Sketch2 (3)" plane through (0, 0, 0) normal (0, 0, 1) x (1, 0, 0) in component "Neogrid - Base Cover 2x1"
  line L0 (0, 0) -> (83.5, 0)
  line L1 (83.5, 0) -> (83.5, 41.5)
  line L2 (83.5, 41.5) -> (0, 41.5)
  line L3 (0, 41.5) -> (0, 0)
  dimension "d148" = 83.5
  dimension "d149" = 41.5
  constraint horizontal L0
  constraint vertical L1
  constraint horizontal L2
  constraint vertical L3
  constraint coincident L0.start L3
  constraint coincident L3.end L0
  measures "d148" horizontal distance of L0.start L0.end
  measures "d149" vertical distance of L0.end L1.end
extrude "Extrude3''" add sketch "Sketch2 (3)" along normal blind 2.25 separate body makes body 36 in component "Neogrid - Base Cover 2x1"
fillet "Fillet2''" radius 3.75 8 edges at (0, 41.5, 1.125) (83.5, 41.5, 1.125) (83.5, 41.5, 1.125) (83.5, 0, 1.125) (83.5, 0, 1.125) (0, 0, 1.125) (0, 0, 1.125) (0, 41.5, 1.125) on bodies 36 in component "Neogrid - Base Cover 2x1"
combine "Combine1''" operation add target body 36 tool bodies 34 35 34 in component "Neogrid - Base Cover 2x1"
move_body "Move1'" bodies 36 to x (1, 0, 0) y (0, 1, 0) z (0, 0, 1) at (460, 190, 0) in component "Neogrid - Base Cover 2x1"
extrude "Extrude1'''" add sketch "Master Dimensions" along normal blind 42 from surface at 100 separate body contours L0 L5 L19 L25 L36 L38 L39 | L9 L19 L25 L27 L36 L39 | L9 L11 L19 L20 L27 L36 L39 | L11 L19 L20 L23 L34 L36 L39 | L9 L11 L12 L16 L19 L20 L27 L36 | L0 L5 L14 L25 L28 L30 L31 | L19 L23 L34 L35 L36 L39 | L11 L12 L16 L19 L20 L23 L34 L36 | L9 L11 L12 L14 L16 L20 L27 L28 | L9 L14 L25 L27 L28 L30 | L2 L7 L19 L35 L36 L37 L39 | L11 L12 L14 L16 L20 L23 L28 L34 | L9 L11 L14 L20 L27 L28 L30 | L11 L14 L20 L23 L28 L30 L34 | L14 L23 L28 L30 L34 L35 | L2 L7 L14 L28 L29 L30 L35 makes body 37
chamfer "Chamfer1'''" distance 1.5 angle 45 4 edges at (20.75, 13.5, 144.25) (20.75, 28, 144.25) (20.75, 13.5, 102.25) (20.75, 28, 102.25) on bodies 37
extrude "Extrude2'''" cut 1 faces at (16.5, 22.1667, 130.25) along direction (1, 0, 0) blind 1 on bodies 37 bodies 37
extrude "Extrude3'''" cut 1 faces at (25, 22.1667, 130.25) along direction (-1, 0, 0) blind 1 on bodies 37 bodies 37
component "Gridfinity bin 1x1x1" placed x (1, 0, 0) y (0, 1, 0) z (0, 0, 1) at (0, 0, 0)
component "Neogrid - Base Cover 2x2" placed x (1, 0, 0) y (0, 1, 0) z (0, 0, 1) at (0, 0, 0)
component "Neogrid - Base Cover 2x1" placed x (1, 0, 0) y (0, 1, 0) z (0, 0, 1) at (0, 0, 0)
equation "d4 = -( 2.15 mm )"
equation "d24 = GridfinityFillet"
equation "GridfinityFillet = 3.75 mm"
equation "d26 = GridfinityFillet"
equation "d27 = GridfinityFillet"
equation "d28 = GridfinityFillet"
equation "NeoGridWidth = 8.5 mm"
equation "d30 = NeoGridWidth / 2"
equation "d31 = NeoGridWidth / 2"
equation "d32 = NeoGridWallThickness"
equation "NeoGridWallThickness = 3 mm"
equation "d34 = NeoGridWallThickness"
equation "NeogridHeight = 21 mm"
equation "d36 = NeogridHeight"
equation "NeogridTopChamfer = 1.5 mm"
equation "NeogridCornerChamfer = 3 mm"
equation "d40 = NeogridCornerChamfer"
equation "d41 = NeogridCornerChamfer"
equation "d42 = NeogridTopChamfer"
equation "d44 = NeogridHeight"
equation "d47 = NeogridHeight - 3 mm"
equation "d49 = NeogridCornerChamfer"
equation "d50 = NeogridTopChamfer"
equation "d51 = NeogridTopChamfer"
equation "d60 = NeogridCornerChamfer"
equation "d61 = NeogridCornerChamfer"
equation "d63 = NeogridTopChamfer"
equation "d64 = NeogridCornerChamfer"
equation "d65 = NeogridTopChamfer"
equation "d66 = NeogridTopChamfer"
equation "d69 = NeogridTopChamfer"
equation "d108 = ( 41.5 * 2 ) * 1 mm"
equation "d110 = ( 41.5 * 3 ) * 1 mm"
equation "d115 = -( 2.15 mm )"
equation "d136 = -( 2.15 mm )"
equation "d155 = NeogridHeight * 2"
equation "d157 = NeogridTopChamfer"
named bodies: "base", "Neogrid - X Junction - Base", "Neogrid - X Junction - Top", "Neogrid - T Junction - Base", "Neogrid - I Junction - Base", "Neogrid - End Cap - Base", "Neogrid - L Junction - Base", "Neogrid - Base Cover 1x1", "Gridfinity Baseline 1x1x1", "Neogrid - L Junction - Top", "Neogrid - I Junction - Top (1)", "Neogrid - T Junction - Top", "Neogrid - I Junction - Top", "Neogrid - Single Label", "Neogrid - Double Label", "Neogrid - Double Trim - Base", "Neogrid - Triple Trim - Base", "Neogrid - Quadruple Trim - Base", "Neogrid - Single Trim - Base", "Gridfinity bin 1x1x1 (2) (1) (1)", "Gridfinity bin 1x1x1 (2) (2) (1)", "Gridfinity bin 1x1x1 (2) (2) (2)", "Gridfinity bin 1x1x1 (2) (3) (1)", "Gridfinity bin 1x1x1 (2) (3) (2)", "Gridfinity bin 1x1x1 (2) (3) (3)", "Neogrid - Double Trim - Top", "Neogrid - Triple Trim - Base (1)", "Neogrid - Quadruple Trim - Base (1)", "base (1)", "base (2)", "base (3)", "Gridfinity bin 2x2x1", "Gridfinity bin 1x2x1"
